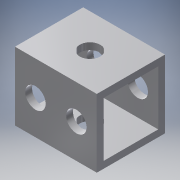
# Autodesk Inventor part: sensor_attach
Saved by Autodesk Inventor 2018 (Build 220112000, 112)
## iProperties
Created: 2018-04-03
Part Number: sensor_attach
Material: アルミニウム 6061
Document SubType Name: Modeling
Designer: NaMACHAN
Density: 2.7 g/cm^3
Appearance: アルミニウム - フラット
Author: NaMACHAN
Autodesk Inventor part; units mm, degrees
ref_plane "YZ Plane" through (0, 0, 0) normal (1, 0, 0) x (0, 1, 0)
ref_plane "XZ Plane" through (0, 0, 0) normal (0, 1, 0) x (-1, 0, 0)
ref_plane "XY Plane" through (0, 0, 0) normal (0, 0, 1) x (1, 0, 0)
sketch "スケッチ1" plane through (0, 0, 0) normal (0, 1, 0) x (-1, 0, 0)
  line L0 (-6, -5) -> (6, -5)
  line L1 (6, -5) -> (6, 5)
  line L2 (6, 5) -> (-6, 5)
  line L3 (-6, 5) -> (-6, -5)
  line L4 (-6, -5) -> (6, 5) construction
  line L5 (6, -5) -> (-6, 5) construction
  point P0 (0, 0)
  dimension "d0" = 12
  dimension "d1" = 10
  constraints: 12 end point, 2 midpoint, 2 parallel, 1 horizontal, 1 perpendicular
  measures "d0" distance of L2.end L1.end
  measures "d1" distance of L1.end L0.end
extrude "押し出し1" add sketch "スケッチ1" along normal blind 10
sketch "スケッチ3" plane through (0, 10, 0) normal (0, 1, 0) x (1, 0, 0)
  line L0 (6, -5) -> (6, 5) projected
  line L1 (-6, 5) -> (-6, -5) projected
  point P0 (0, 0)
  point P1 (3, 0)
  point P2 (-3, 0)
  point P3 (-6, 0)
  dimension "d4" = 3
  dimension "d12" = 3
  constraints: 2 horizontal alignment, 1 midpoint
  measures "d4" distance from line of L0 point (3, 0)
  measures "d12" distance from line of L1 point (-3, 0)
hole "穴1" at (3, 10, 0) at (-3, 10, 0) direction (0, -1, 0) diameter 3 end through all
sketch "スケッチ4" plane through (6, 0, -5) normal (0, 0, -1) x (-1, 0, 0)
  line L0 (0, 0) -> (12, 0) projected
  line L1 (12, 0) -> (12, 10) projected
  point P0 (6, 0)
  point P1 (6, 5)
  point P2 (6, 0)
  point P3 (12, 5)
  constraints: 2 midpoint, 1 horizontal alignment, 1 vertical alignment
hole "穴2" at (0, 5, -5) direction (0, 0, 1) diameter 3 end through all
sketch "スケッチ5" plane through (6, 0, 5) normal (1, 0, 0) x (0, 0, -1)
  line L0 (1, 1) -> (9, 1)
  line L1 (9, 1) -> (9, 9)
  line L2 (9, 9) -> (1, 9)
  line L3 (1, 9) -> (1, 1)
  line L4 (1, 1) -> (9, 9) construction
  line L5 (9, 1) -> (1, 9) construction
  line L6 (10, 0) -> (10, 10) projected
  point P0 (5, 0)
  point P1 (5, 5)
  point P2 (5, 5)
  point P3 (5, 5)
  point P4 (10, 5)
  dimension "d20" = 8
  dimension "d21" = 8
  constraints: 12 end point, 5 midpoint, 2 parallel, 1 horizontal, 1 horizontal alignment, 1 perpendicular, 1 vertical alignment
  measures "d20" distance of L0.end L1.end
  measures "d21" distance of L0.start L0.end
extrude "押し出し2" cut sketch "スケッチ5" against normal blind 12
